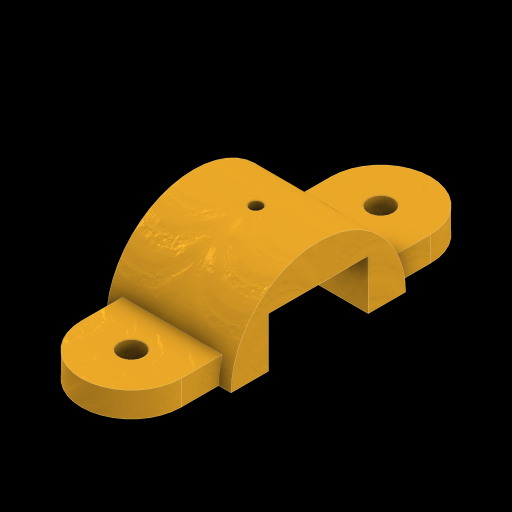
# Autodesk Inventor part: ANS7S-TUT-BK
Saved by Autodesk Inventor 2024 (Build 280153000, 153)
## iProperties
Created: 2023-10-14
Part Number: ANS7S-TUT-BK
Material: Brass, Soft Yellow, Welded
Document SubType Name: Modeling
Designer: bennk
Mass: 119.569 g
Surface Area: 288.689 cm^2
Volume: 119.772 cm^3
Density: 8.5 g/cm^3
Appearance: Weld - Brass
Author: bennk
Autodesk Inventor part; units mm, degrees
ref_plane "YZ Plane" through (0, 0, 0) normal (1, 0, 0) x (0, 1, 0)
ref_plane "XZ Plane" through (0, 0, 0) normal (0, 1, 0) x (-1, 0, 0)
ref_plane "XY Plane" through (0, 0, 0) normal (0, 0, 1) x (1, 0, 0)
sketch "Sketch1" plane through (0, 0, 0) normal (0, 1, 0) x (-1, 0, 0)
  line L0 (0, 88.9) -> (0, -88.9) construction
  line L1 (25.4, 63.5) -> (25.4, -63.5)
  line L2 (-25.4, -63.5) -> (-25.4, 63.5)
  arc A0 (25.4, 63.5) -> (-25.4, 63.5) centre (0, 63.5) ccw
  arc A1 (-25.4, -63.5) -> (25.4, -63.5) centre (0, -63.5) ccw
  circle A2 centre (0, 63.5) radius 6.35
  circle A3 centre (0, -63.5) radius 6.35
  point P0 (0, 0)
  point P1 (0, 0)
  dimension "d0" = 127
  dimension "d1" = 12.7
  dimension "d2" = 12.7
  dimension "d3" = 25.4
  constraints: 8 end point, 6 point on circle, 4 centre point, 4 tangent, 3 coincident, 2 point on line, 1 midpoint, 1 parallel, 1 vertical
  measures "d0" distance of A1.centre A0.centre
  measures "d1" diameter of A2
  measures "d2" diameter of A3
  measures "d3" radius of A1
extrude "BASE" add sketch "Sketch1" along normal blind 12.7
sketch "Sketch2" plane through (0, 0, 0) normal (1, 0, 0) x (0, 1, 0)
  arc A0 (0, -44.45) -> (0, 44.45) centre (0, 0) ccw
  arc A1 (0, -31.75) -> (0, 31.75) centre (0, 0) ccw
  line L0 (0, -63.5) -> (0, 63.5) projected
  line L1 (0, 31.75) -> (15.875, 31.75)
  line L2 (15.875, 31.75) -> (15.875, -31.75)
  line L3 (15.875, -31.75) -> (0, -31.75)
  line L4 (0, -31.75) -> (0, 31.75)
  line L5 (0, 63.5) -> (0, -63.5) projected
  point P0 (7.9375, -31.75)
  point P1 (0, 0)
  point P2 (15.875, -27.4963)
  point P3 (15.875, 27.4963)
  point P4 (0, -31.75)
  dimension "d7" = 44.45
  dimension "d8" = 31.75
  dimension "d16" = 63.5
  dimension "d17" = 31.75
  dimension "d18" = 15.875
  constraints: 8 end point, 5 point on line, 4 point on circle, 2 centre point, 2 coincident, 2 parallel, 1 horizontal, 1 midpoint, 1 perpendicular, 2 other
  measures "d7" radius of A0
  measures "d8" radius of A1
  measures "d16" distance from line of point (7.938, -31.75) L1
  measures "d17" distance from line of point (0, 0) L1
  measures "d18" distance between parallel lines of L0 L2
extrude "REMOVED CENTER OF BASE" cut sketch "Sketch2" along normal through all both and the other way through all
extrude "ARCH" add sketch "Sketch2" along normal mid plane 63.5
sketch "Sketch3" plane through (0, 0, 0) normal (0, 1, 0) x (-1, 0, 0)
  circle A0 centre (0, 0) radius 3.175
  dimension "d13" = 6.35
  constraints: 1 centre point, 1 coincident
  measures "d13" diameter of A0
extrude "TOPHOLE" cut sketch "Sketch3" along normal through all
sketch "Sketch5" plane through (31.75, 0, 0) normal (1, 0, 0) x (0, 0, -1)
  line L0 (-44.45, 0) -> (44.45, 0) projected
  circle A0 centre (0, 0) radius 31.75
  point P0 (-31.75, 0)
  dimension "d26" = 31.75
  constraints: 1 coincident, 1 horizontal alignment, 2 other
extrude "CIRCULAR" [suppressed]
sketch "Sketch6" plane through (31.75, 0, 0) normal (1, 0, 0) x (0, 0, -1)
  line L0 (-25.4, 25.4) -> (25.4, 25.4)
  line L1 (25.4, 25.4) -> (25.4, 0)
  line L2 (25.4, 0) -> (-25.4, 0)
  line L3 (-25.4, 0) -> (-25.4, 25.4)
  point P0 (0, 0)
  point P1 (0, 0)
  point P2 (0, 0)
  dimension "d23" = 50.8
  dimension "d24" = 25.4
  dimension "d25" = 25.4
  constraints: 8 end point, 2 parallel, 1 horizontal, 1 midpoint, 1 perpendicular
  measures "d23" distance between parallel lines of L1 L3
  measures "d24" distance from line of point (0, 0) L3
  measures "d25" distance between parallel lines of L0 L2
extrude "SQUARE" cut sketch "Sketch6" against normal through all
equation "\"d2\" = d1"
equation "\"d17\" = 0.5 * d16"
equation "\"d11\" = d16"
equation "\"d24\" = 0.5 * d23"
body "Solid1"
